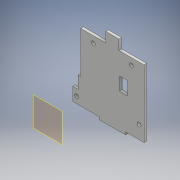
# Autodesk Inventor part: arm_2_case
Saved by Autodesk Inventor 2018 (Build 220112000, 112)
## iProperties
Created: 2018-02-08
Part Number: arm_2_case
Material: Genérico
Document SubType Name: Modeling
Designer: se_ma
Density: 1 g/cm^3
Appearance: Valor por defecto
Author: se_ma
Autodesk Inventor part; units mm, degrees
ref_plane "YZ Plane" through (0, 0, 0) normal (1, 0, 0) x (0, 1, 0)
ref_plane "XZ Plane" through (0, 0, 0) normal (0, 1, 0) x (-1, 0, 0)
ref_plane "XY Plane" through (0, 0, 0) normal (0, 0, 1) x (1, 0, 0)
sketch "Boceto1" plane through (0, 0, 0) normal (0, 1, 0) x (-1, 0, 0)
  line L0 (48, 0) -> (48, -51)
  line L1 (48, -51) -> (0, -51)
  line L2 (0, -51) -> (0, 0)
  line L3 (24, 7.5) -> (29, 7.5)
  line L4 (29, 7.5) -> (29, 0)
  line L5 (24, 7.5) -> (19, 7.5)
  line L6 (19, 7.5) -> (19, 0)
  line L7 (24, 7.5) -> (24, -1.25)
  circle A0 centre (24, -1.25) radius 1.5
  line L8 (29, 0) -> (48, 0)
  line L9 (19, 0) -> (0, 0)
  dimension "d0" = 48
  dimension "d1" = 51
  dimension "d3" = 5
  dimension "d4" = 5
  dimension "d5" = 8.75
  dimension "d6" = 3
  constraints: 20 end point, 2 equal length, 1 centre point, 1 coincident, 1 horizontal, 1 point on line, 1 vertical
  measures "d0" distance of L0.end L1.end
  measures "d1" distance of L0.start L0.end
  measures "d3" distance of L3.start L3.end
  measures "d4" distance of L3.start L5.end
  measures "d5" distance of L3.start L7.end
  measures "d6" diameter of A0
extrude "Extrusión1" add sketch "Boceto1" along normal blind 2
ref_plane "Plano de trabajo1" through (-48, -25, -47.5) normal (0, -1, 0) x (1, 0, 0)
sketch "Boceto4" plane through (0, 2, 0) normal (0, 1, 0) x (1, 0, 0)
  line L0 (0, 51) -> (-48, 51) projected
  line L1 (-24, 51) -> (-24, 53)
  line L2 (-24, 53) -> (-34, 53)
  line L3 (-34, 53) -> (-34, 51)
  line L4 (-34, 51) -> (-14, 51)
  line L5 (-14, 51) -> (-14, 53)
  line L6 (-14, 53) -> (-24, 53)
  point P0 (0, 0)
  dimension "d18" = 2
  dimension "d19" = 10
  dimension "d20" = 20
  constraints: 12 end point, 5 perpendicular, 2 point on line, 1 midpoint, 1 vertical
  measures "d18" distance of L1.start L1.end
  measures "d19" distance of L1.end L2.end
  measures "d20" distance of L3.end L4.end
extrude "Extrusión4" add sketch "Boceto4" against normal blind 2
sketch "Boceto6" plane through (0, 2, 0) normal (0, 1, 0) x (1, 0, 0)
  line L0 (-48, 47.5) -> (-48, 31.5) projected
  line L1 (-48, 47.5) -> (-18.5, 47.5)
  line L2 (-18.5, 47.5) -> (-18.5, 26.5)
  line L3 (-18.5, 26.5) -> (-18.5, 16.5)
  line L4 (-18.5, 16.5) -> (-12.5, 16.5)
  line L5 (-12.5, 16.5) -> (-12.5, 26.5)
  line L6 (-12.5, 26.5) -> (-18.5, 26.5)
  point P0 (0, 0)
  dimension "d26" = 29.5
  dimension "d27" = 21
  dimension "d28" = 10
  dimension "d29" = 6
  constraints: 12 end point, 4 perpendicular, 1 horizontal, 1 vertical
  measures "d26" distance of L0.start L1.end
  measures "d27" distance of L1.end L2.end
  measures "d28" distance of L2.end L3.end
  measures "d29" distance of L3.end L4.end
extrude "Extrusión6" cut sketch "Boceto6" against normal blind 2
sketch "Boceto7" plane through (0, 2, 0) normal (0, 1, 0) x (1, 0, 0)
  circle A0 centre (-24, 1.25) radius 1.5 projected
  circle A1 centre (-24, 1.25) radius 1.5
  point P0 (0, 0)
  constraints: 1 centre point, 1 coincident
extrude "Extrusión7" add sketch "Boceto7" against normal blind 2
sketch "Boceto8" plane through (0, 2, 0) normal (0, 1, 0) x (1, 0, 0)
  line L0 (-48, 51) -> (-48, 0) projected
  line L1 (-48, 51) -> (-48, 31.5)
  line L2 (-48, 31.5) -> (-50, 31.5)
  line L3 (-50, 31.5) -> (-50, 41)
  line L4 (-50, 41) -> (-54, 41)
  line L5 (-54, 41) -> (-54, 51)
  line L6 (-54, 51) -> (-48, 51)
  point P0 (0, 0)
  dimension "d34" = 19.5
  dimension "d35" = 2
  dimension "d36" = 9.5
  dimension "d37" = 4
  constraints: 12 end point, 3 perpendicular, 1 horizontal, 1 parallel, 1 point on line
  measures "d34" distance of L0.start L1.end
  measures "d35" distance of L1.end L2.end
  measures "d36" distance of L2.end L3.end
  measures "d37" distance of L3.end L4.end
extrude "Extrusión8" add sketch "Boceto8" against normal blind 2
sketch "Boceto9" plane through (0, 2, 0) normal (0, 1, 0) x (1, 0, 0)
  line L0 (-48, 0) -> (-29, 0) projected
  line L1 (-48, 0) -> (-48, 5)
  line L2 (-48, 31.5) -> (-48, 0) projected
  line L3 (-48, 5) -> (-38.5, 5)
  line L4 (-48, 5) -> (-9.5, 5)
  circle A0 centre (-38.5, 5) radius 1.5
  circle A1 centre (-9.5, 5) radius 1.5
  line L5 (0, 51) -> (-14, 51) projected
  line L6 (0, 51) -> (0, 41)
  line L7 (0, 0) -> (0, 51) projected
  line L8 (0, 41) -> (-3.75, 41)
  circle A2 centre (-3.75, 41) radius 1.5
  line L9 (-34, 51) -> (-54, 51) projected
  line L10 (-54, 51) -> (-51, 51)
  line L11 (-51, 51) -> (-51, 46)
  circle A3 centre (-51, 46) radius 1.5
  dimension "d40" = 5
  dimension "d41" = 9.5
  dimension "d42" = 38.5
  dimension "d43" = 3
  dimension "d44" = 3
  dimension "d45" = 10
  dimension "d46" = 3.75
  dimension "d47" = 3
  dimension "d48" = 3
  dimension "d49" = 3
  constraints: 14 end point, 4 centre point, 4 coincident, 3 point on line, 2 horizontal, 2 perpendicular
  measures "d40" distance of L0.start L1.end
  measures "d41" distance of L1.end L3.end
  measures "d42" distance of L1.end L4.end
  measures "d43" diameter of A0
  measures "d44" diameter of A1
  measures "d45" distance of L5.start L6.end
  measures "d46" distance of L6.end L8.end
  measures "d47" diameter of A2
  measures "d48" distance of L9.end L10.end
  measures "d49" diameter of A3
extrude "Extrusión9" cut sketch "Boceto9" against normal blind 2
